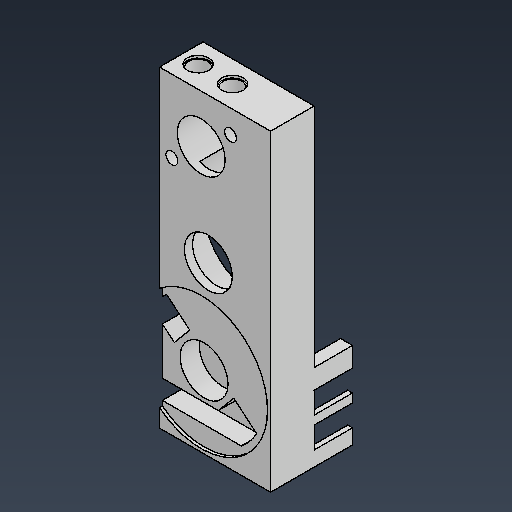
# Autodesk Inventor part: Left_gearbox
Saved by Autodesk Inventor 2026.2 (Build 302298010, 298A)
## iProperties
Created: 2026-04-03
Part Number: Left_gearbox
Material: Generic
Document SubType Name: Modeling
Designer: szymo
Density: 1 g/cm^3
Appearance: Default
Author: szymo
Autodesk Inventor part; units mm, degrees
(part 1 of 2)
ref_plane "YZ Plane" through (0, 0, 0) normal (1, 0, 0) x (0, 1, 0)
ref_plane "XZ Plane" through (0, 0, 0) normal (0, 1, 0) x (-1, 0, 0)
ref_plane "XY Plane" through (0, 0, 0) normal (0, 0, 1) x (1, 0, 0)
ref_plane "Work Plane3" through (-33.4195, -4.4195, -0.6) normal (0, 0, -1) x (-0.5, 0.8660254, 0)
ref_plane "Work Plane4" through (-33.7893, 35.5042, 0.6) normal (0, 0, -1) x (-0.5735764, 0.819152, 0)
sketch "Sketch2" plane through (0, 0, 0) normal (0, 0, 1) x (1, 0, 0)
  circle A0 centre (-8.3716, 60.4381) radius 1.0564 construction
  circle A1 centre (-20.6284, 50.1535) radius 1.0564 construction
  circle A2 centre (-14.5, 55.2958) radius 5
  circle A3 centre (-14.5, 55.2958) radius 13.85 construction
  circle A4 centre (-8.9947, 46.9477) radius 1.25 construction
  arc A5 (-11.5285, 53.3387) -> (-12.3283, 54.22) centre (-15.6066, 50.4414) ccw construction
  arc A6 (-11.1905, 53.4626) -> (-11.5285, 53.3387) centre (-8.9947, 46.9477) ccw construction
  arc A7 (-11.1496, 54.652) -> (-11.1905, 53.4626) centre (-6.206, 53.8864) ccw construction
  arc A8 (-10.7434, 54.7542) -> (-11.1496, 54.652) centre (-8.9947, 46.9477) ccw construction
  arc A9 (-10.1443, 53.7259) -> (-10.7434, 54.7542) centre (-14.7357, 51.7398) ccw construction
  arc A10 (-9.788, 53.7767) -> (-10.1443, 53.7259) centre (-8.9947, 46.9477) ccw construction
  arc A11 (-9.5007, 54.9316) -> (-9.788, 53.7767) centre (-4.8243, 53.1549) ccw construction
  arc A12 (-9.0821, 54.9472) -> (-9.5007, 54.9316) centre (-8.9947, 46.9477) ccw construction
  arc A13 (-8.7099, 53.8168) -> (-9.0821, 54.9472) centre (-13.6139, 52.8287) ccw construction
  arc A14 (-8.3508, 53.7924) -> (-8.7099, 53.8168) centre (-8.9947, 46.9477) ccw construction
  arc A15 (-7.8296, 54.8624) -> (-8.3508, 53.7924) centre (-3.6248, 52.1522) ccw construction
  arc A16 (-7.417, 54.7905) -> (-7.8296, 54.8624) centre (-8.9947, 46.9477) ccw construction
  arc A17 (-7.288, 53.6074) -> (-7.417, 54.7905) centre (-12.2903, 53.6605) ccw construction
  arc A18 (-6.9418, 53.509) -> (-7.288, 53.6074) centre (-8.9947, 46.9477) ccw construction
  arc A19 (-6.2095, 54.4472) -> (-6.9418, 53.509) centre (-2.6601, 50.922) ccw construction
  arc A20 (-5.8209, 54.2911) -> (-6.2095, 54.4472) centre (-8.9947, 46.9477) ccw construction
  arc A21 (-5.9406, 53.1071) -> (-5.8209, 54.2911) centre (-10.8226, 54.199) ccw construction
  arc A22 (-5.6225, 52.9388) -> (-5.9406, 53.1071) centre (-8.9947, 46.9477) ccw construction
  arc A23 (-4.7112, 53.7042) -> (-5.6225, 52.9388) centre (-1.9722, 49.5181) ccw construction
  arc A24 (-4.3634, 53.4708) -> (-4.7112, 53.7042) centre (-8.9947, 46.9477) ccw construction
  arc A25 (-4.7268, 52.3375) -> (-4.3634, 53.4708) centre (-9.275, 54.4206) ccw construction
  arc A26 (-4.4505, 52.1067) -> (-4.7268, 52.3375) centre (-8.9947, 46.9477) ccw construction
  arc A27 (-3.4, 52.666) -> (-4.4505, 52.1067) centre (-1.5913, 48.0019) ccw construction
  arc A28 (-3.1084, 52.3653) -> (-3.4, 52.666) centre (-8.9947, 46.9477) ccw construction
  arc A29 (-3.6994, 51.3323) -> (-3.1084, 52.3653) centre (-7.7151, 54.3155) ccw construction
  arc A30 (-3.4772, 51.0492) -> (-3.6994, 51.3323) centre (-8.9947, 46.9477) ccw construction
  arc A31 (-2.3334, 51.3778) -> (-3.4772, 51.0492) centre (-1.5339, 46.4396) ccw construction
  arc A32 (-2.1106, 51.0231) -> (-2.3334, 51.3778) centre (-8.9947, 46.9477) ccw construction
  arc A33 (-2.9035, 50.1356) -> (-2.1106, 51.0231) centre (-6.2112, 53.8885) ccw construction
  arc A34 (-2.745, 49.8124) -> (-2.9035, 50.1356) centre (-8.9947, 46.9477) ccw construction
  arc A35 (-1.5579, 49.896) -> (-2.745, 49.8124) centre (-1.8025, 44.8995) ccw construction
  arc A36 (-1.4137, 49.5027) -> (-1.5579, 49.896) centre (-8.9947, 46.9477) ccw construction
  arc A37 (-2.3738, 48.7995) -> (-1.4137, 49.5027) centre (-4.829, 53.1581) ccw construction
  arc A38 (-2.286, 48.4504) -> (-2.3738, 48.7995) centre (-8.9947, 46.9477) ccw construction
  arc A39 (-1.1074, 48.2854) -> (-2.286, 48.4504) centre (-2.3855, 43.4489) ccw construction
  arc A40 (-1.0482, 47.8707) -> (-1.1074, 48.2854) centre (-8.9947, 46.9477) ccw construction
  arc A41 (-2.1335, 47.3824) -> (-1.0482, 47.8707) centre (-3.6288, 52.1563) ccw construction
  arc A42 (-2.1202, 47.0227) -> (-2.1335, 47.3824) centre (-8.9947, 46.9477) ccw construction
  arc A43 (-1.0016, 46.6163) -> (-2.1202, 47.0227) centre (-3.2574, 42.1512) ccw construction
  arc A44 (-1.0299, 46.1984) -> (-1.0016, 46.6163) centre (-8.9947, 46.9477) ccw construction
  arc A45 (-2.193, 45.9464) -> (-1.0299, 46.1984) centre (-2.6631, 50.9268) ccw construction
  arc A46 (-2.2548, 45.5918) -> (-2.193, 45.9464) centre (-8.9947, 46.9477) ccw construction
  arc A47 (-1.2452, 44.9616) -> (-2.2548, 45.5918) centre (-4.38, 41.0632) ccw construction
  arc A48 (-1.3597, 44.5588) -> (-1.2452, 44.9616) centre (-8.9947, 46.9477) ccw construction
  arc A49 (-2.5499, 44.5541) -> (-1.3597, 44.5588) centre (-1.9742, 49.5234) ccw construction
  arc A50 (-2.684, 44.2201) -> (-2.5499, 44.5541) centre (-8.9947, 46.9477) ccw construction
  arc A51 (-1.8274, 43.3938) -> (-2.684, 44.2201) centre (-5.7043, 40.2323) ccw construction
  arc A52 (-2.0233, 43.0236) -> (-1.8274, 43.3938) centre (-8.9947, 46.9477) ccw construction
  arc A53 (-3.1883, 43.2665) -> (-2.0233, 43.0236) centre (-1.5921, 48.0075) ccw construction
  arc A54 (-3.3889, 42.9676) -> (-3.1883, 43.2665) centre (-8.9947, 46.9477) ccw construction
  arc A55 (-2.723, 41.9813) -> (-3.3889, 42.9676) centre (-7.1724, 39.6949) ccw construction
  arc A56 (-2.9915, 41.6599) -> (-2.723, 41.9813) centre (-8.9947, 46.9477) ccw construction
  arc A57 (-4.0806, 42.1397) -> (-2.9915, 41.6599) centre (-1.5335, 46.4452) ccw construction
  arc A58 (-4.3389, 41.8891) -> (-4.0806, 42.1397) centre (-8.9947, 46.9477) ccw construction
  arc A59 (-3.8926, 40.7858) -> (-4.3389, 41.8891) centre (-8.7202, 39.4745) ccw construction
  arc A60 (-4.2221, 40.5273) -> (-3.8926, 40.7858) centre (-8.9947, 46.9477) ccw construction
  arc A61 (-5.1876, 41.223) -> (-4.2221, 40.5273) centre (-1.801, 44.9049) ccw construction
  arc A62 (-5.4924, 41.0316) -> (-5.1876, 41.223) centre (-8.9947, 46.9477) ccw construction
  arc A63 (-5.2852, 39.8597) -> (-5.4924, 41.0316) centre (-10.2799, 39.5808) ccw construction
  arc A64 (-5.6612, 39.6753) -> (-5.2852, 39.8597) centre (-8.9947, 46.9477) ccw construction
  arc A65 (-6.461, 40.5566) -> (-5.6612, 39.6753) centre (-2.3829, 43.4539) ccw construction
  arc A66 (-6.799, 40.4327) -> (-6.461, 40.5566) centre (-8.9947, 46.9477) ccw construction
  arc A67 (-6.8399, 39.2433) -> (-6.799, 40.4327) centre (-11.7835, 40.0089) ccw construction
  arc A68 (-7.2461, 39.1411) -> (-6.8399, 39.2433) centre (-8.9947, 46.9477) ccw construction
  arc A69 (-7.8452, 40.1695) -> (-7.2461, 39.1411) centre (-3.2538, 42.1556) ccw construction
  arc A70 (-8.2015, 40.1186) -> (-7.8452, 40.1695) centre (-8.9947, 46.9477) ccw construction
  arc A71 (-8.4888, 38.9637) -> (-8.2015, 40.1186) centre (-13.1652, 40.7404) ccw construction
  arc A72 (-8.9074, 38.9481) -> (-8.4888, 38.9637) centre (-8.9947, 46.9477) ccw construction
  arc A73 (-9.2795, 40.0786) -> (-8.9074, 38.9481) centre (-4.3756, 41.0667) ccw construction
  arc A74 (-9.6387, 40.1029) -> (-9.2795, 40.0786) centre (-8.9947, 46.9477) ccw construction
  arc A75 (-10.1598, 39.033) -> (-9.6387, 40.1029) centre (-14.3646, 41.7431) ccw construction
  arc A76 (-10.5725, 39.1048) -> (-10.1598, 39.033) centre (-8.9947, 46.9477) ccw construction
  arc A77 (-10.7015, 40.2879) -> (-10.5725, 39.1048) centre (-5.6992, 40.2348) ccw construction
  arc A78 (-11.0477, 40.3863) -> (-10.7015, 40.2879) centre (-8.9947, 46.9477) ccw construction
  arc A79 (-11.7799, 39.4481) -> (-11.0477, 40.3863) centre (-15.3294, 42.9733) ccw construction
  arc A80 (-12.1686, 39.6042) -> (-11.7799, 39.4481) centre (-8.9947, 46.9477) ccw construction
  arc A81 (-12.0488, 40.7883) -> (-12.1686, 39.6042) centre (-7.1669, 39.6963) ccw construction
  arc A82 (-12.367, 40.9565) -> (-12.0488, 40.7883) centre (-8.9947, 46.9477) ccw construction
  arc A83 (-13.2783, 40.1911) -> (-12.367, 40.9565) centre (-16.0173, 44.3772) ccw construction
  arc A84 (-13.6261, 40.4246) -> (-13.2783, 40.1911) centre (-8.9947, 46.9477) ccw construction
  arc A85 (-13.2627, 41.5578) -> (-13.6261, 40.4246) centre (-8.7145, 39.4747) ccw construction
  arc A86 (-13.5389, 41.7886) -> (-13.2627, 41.5578) centre (-8.9947, 46.9477) ccw construction
  arc A87 (-14.5895, 41.2294) -> (-13.5389, 41.7886) centre (-16.3982, 45.8935) ccw construction
  arc A88 (-14.8811, 41.53) -> (-14.5895, 41.2294) centre (-8.9947, 46.9477) ccw construction
  arc A89 (-14.29, 42.563) -> (-14.8811, 41.53) centre (-10.2743, 39.5798) ccw construction
  arc A90 (-14.5123, 42.8461) -> (-14.29, 42.563) centre (-8.9947, 46.9477) ccw construction
  arc A91 (-15.6561, 42.5175) -> (-14.5123, 42.8461) centre (-16.4556, 47.4558) ccw construction
  arc A92 (-15.8788, 42.8722) -> (-15.6561, 42.5175) centre (-8.9947, 46.9477) ccw construction
  arc A93 (-15.086, 43.7598) -> (-15.8788, 42.8722) centre (-11.7782, 40.0068) ccw construction
  arc A94 (-15.2445, 44.0829) -> (-15.086, 43.7598) centre (-8.9947, 46.9477) ccw construction
  arc A95 (-16.4316, 43.9993) -> (-15.2445, 44.0829) centre (-16.187, 48.9959) ccw construction
  arc A96 (-16.5757, 44.3926) -> (-16.4316, 43.9993) centre (-8.9947, 46.9477) ccw construction
  arc A97 (-15.6157, 45.0959) -> (-16.5757, 44.3926) centre (-13.1605, 40.7372) ccw construction
  arc A98 (-15.7035, 45.4449) -> (-15.6157, 45.0959) centre (-8.9947, 46.9477) ccw construction
  arc A99 (-16.8821, 45.61) -> (-15.7035, 45.4449) centre (-15.6039, 50.4465) ccw construction
  arc A100 (-16.9413, 46.0246) -> (-16.8821, 45.61) centre (-8.9947, 46.9477) ccw construction
  arc A101 (-15.856, 46.5129) -> (-16.9413, 46.0246) centre (-14.3607, 41.739) ccw construction
  arc A102 (-15.8693, 46.8726) -> (-15.856, 46.5129) centre (-8.9947, 46.9477) ccw construction
  arc A103 (-16.9879, 47.2791) -> (-15.8693, 46.8726) centre (-14.7321, 51.7441) ccw construction
  arc A104 (-16.9596, 47.6969) -> (-16.9879, 47.2791) centre (-8.9947, 46.9477) ccw construction
  arc A105 (-15.7964, 47.9489) -> (-16.9596, 47.6969) centre (-15.3264, 42.9685) ccw construction
  arc A106 (-15.7347, 48.3035) -> (-15.7964, 47.9489) centre (-8.9947, 46.9477) ccw construction
  arc A107 (-16.7443, 48.9337) -> (-15.7347, 48.3035) centre (-13.6095, 52.8322) ccw construction
  arc A108 (-16.6297, 49.3365) -> (-16.7443, 48.9337) centre (-8.9947, 46.9477) ccw construction
  arc A109 (-15.4396, 49.3412) -> (-16.6297, 49.3365) centre (-16.0153, 44.3719) ccw construction
  arc A110 (-15.3055, 49.6752) -> (-15.4396, 49.3412) centre (-8.9947, 46.9477) ccw construction
  arc A111 (-16.162, 50.5015) -> (-15.3055, 49.6752) centre (-12.2852, 53.663) ccw construction
  arc A112 (-15.9662, 50.8717) -> (-16.162, 50.5015) centre (-8.9947, 46.9477) ccw construction
  arc A113 (-14.8012, 50.6289) -> (-15.9662, 50.8717) centre (-16.3974, 45.8878) ccw construction
  arc A114 (-14.6005, 50.9277) -> (-14.8012, 50.6289) centre (-8.9947, 46.9477) ccw construction
  arc A115 (-15.2665, 51.914) -> (-14.6005, 50.9277) centre (-10.817, 54.2004) ccw construction
  arc A116 (-14.998, 52.2355) -> (-15.2665, 51.914) centre (-8.9947, 46.9477) ccw construction
  arc A117 (-13.9089, 51.7556) -> (-14.998, 52.2355) centre (-16.456, 47.4501) ccw construction
  arc A118 (-13.6505, 52.0062) -> (-13.9089, 51.7556) centre (-8.9947, 46.9477) ccw construction
  arc A119 (-14.0969, 53.1095) -> (-13.6505, 52.0062) centre (-9.2693, 54.4208) ccw construction
  arc A120 (-13.7674, 53.368) -> (-14.0969, 53.1095) centre (-8.9947, 46.9477) ccw construction
  arc A121 (-12.8019, 52.6723) -> (-13.7674, 53.368) centre (-16.1885, 48.9904) ccw construction
  arc A122 (-12.4971, 52.8637) -> (-12.8019, 52.6723) centre (-8.9947, 46.9477) ccw construction
  arc A123 (-12.7043, 54.0356) -> (-12.4971, 52.8637) centre (-7.7095, 54.3146) ccw construction
  arc A124 (-12.3283, 54.22) -> (-12.7043, 54.0356) centre (-8.9947, 46.9477) ccw construction
  circle A125 centre (-13, 35.0012) radius 5
  arc A126 (-19.3741, 42.1797) -> (-18.7931, 40.8751) centre (-13.6387, 43.9522) ccw construction
  arc A127 (-18.7931, 40.8751) -> (-19.0926, 40.5639) centre (-13, 35.0012) ccw construction
  arc A128 (-19.0926, 40.5639) -> (-20.4186, 41.0942) centre (-21.969, 35.2948) ccw construction
  arc A129 (-20.4186, 41.0942) -> (-20.7273, 40.6976) centre (-13, 35.0012) ccw construction
  arc A130 (-20.7273, 40.6976) -> (-19.8878, 39.5423) centre (-15.4858, 43.6238) ccw construction
  arc A131 (-19.8878, 39.5423) -> (-20.116, 39.1756) centre (-13, 35.0012) ccw construction
  arc A132 (-20.116, 39.1756) -> (-21.5233, 39.4186) centre (-21.8341, 33.4236) ccw construction
  arc A133 (-21.5233, 39.4186) -> (-21.7428, 38.9665) centre (-13, 35.0012) ccw construction
  arc A134 (-21.7428, 38.9665) -> (-20.6814, 38.011) centre (-17.2242, 42.9186) ccw construction
  arc A135 (-20.6814, 38.011) -> (-20.8284, 37.6049) centre (-13, 35.0012) ccw construction
  arc A136 (-20.8284, 37.6049) -> (-22.2555, 37.55) centre (-21.313, 31.6214) ccw construction
  arc A137 (-22.2555, 37.55) -> (-22.3762, 37.0621) centre (-13, 35.0012) ccw construction
  arc A138 (-22.3762, 37.0621) -> (-21.1393, 36.3482) centre (-18.778, 41.8673) ccw construction
  arc A139 (-21.1393, 36.3482) -> (-21.1986, 35.9204) centre (-13, 35.0012) ccw construction
  arc A140 (-21.1986, 35.9204) -> (-22.5831, 35.57) centre (-20.4287, 29.9669) ccw construction
  arc A141 (-22.5831, 35.57) -> (-22.5998, 35.0677) centre (-13, 35.0012) ccw construction
  arc A142 (-22.5998, 35.0677) -> (-21.2415, 34.6265) centre (-20.0793, 40.516) ccw construction
  arc A143 (-21.2415, 34.6265) -> (-21.2106, 34.1957) centre (-13, 35.0012) ccw construction
  arc A144 (-21.2106, 34.1957) -> (-22.492, 33.5651) centre (-19.2196, 28.5324) ccw construction
  arc A145 (-22.492, 33.5651) -> (-22.4038, 33.0703) centre (-13, 35.0012) ccw construction
  arc A146 (-22.4038, 33.0703) -> (-20.9835, 32.9212) centre (-21.0712, 38.9236) ccw construction
  arc A147 (-20.9835, 32.9212) -> (-20.8637, 32.5062) centre (-13, 35.0012) ccw construction
  arc A148 (-20.8637, 32.5062) -> (-21.986, 31.623) centre (-17.7388, 27.3806) ccw construction
  arc A149 (-21.986, 31.623) -> (-21.7969, 31.1574) centre (-13, 35.0012) ccw construction
  arc A150 (-21.7969, 31.1574) -> (-20.3766, 31.3068) centre (-21.7103, 37.1598) ccw construction
  arc A151 (-20.3766, 31.3068) -> (-20.1731, 30.9258) centre (-13, 35.0012) ccw construction
  arc A152 (-20.1731, 30.9258) -> (-21.0873, 29.8285) centre (-16.0508, 26.5619) ccw construction
  arc A153 (-21.0873, 29.8285) -> (-20.8055, 29.4124) centre (-13, 35.0012) ccw construction
  arc A154 (-20.8055, 29.4124) -> (-19.4473, 29.8538) centre (-21.9688, 35.3016) ccw construction
  arc A155 (-19.4473, 29.8538) -> (-19.169, 29.5235) centre (-13, 35.0012) ccw construction
  arc A156 (-19.169, 29.5235) -> (-19.8351, 28.2601) centre (-14.2295, 26.112) ccw construction
  arc A157 (-19.8351, 28.2601) -> (-19.4729, 27.9117) centre (-13, 35.0012) ccw construction
  arc A158 (-19.4729, 27.9117) -> (-18.2362, 28.6259) centre (-21.8352, 33.4304) ccw construction
  arc A159 (-18.2362, 28.6259) -> (-17.8953, 28.3605) centre (-13, 35.0012) ccw construction
  arc A160 (-17.8953, 28.3605) -> (-18.2842, 26.9864) centre (-12.3545, 26.0506) ccw construction
  arc A161 (-18.2842, 26.9864) -> (-17.8575, 26.7208) centre (-13, 35.0012) ccw construction
  arc A162 (-17.8575, 26.7208) -> (-16.7962, 27.6765) centre (-21.3156, 31.6277) ccw construction
  arc A163 (-16.7962, 27.6765) -> (-16.4077, 27.4879) centre (-13, 35.0012) ccw construction
  arc A164 (-16.4077, 27.4879) -> (-16.5023, 26.0629) centre (-10.5077, 26.3804) ccw construction
  arc A165 (-16.5023, 26.0629) -> (-16.0297, 25.8918) centre (-13, 35.0012) ccw construction
  arc A166 (-16.0297, 25.8918) -> (-15.1904, 27.0473) centre (-20.4325, 29.9725) ccw construction
  arc A167 (-15.1904, 27.0473) -> (-14.7711, 26.9436) centre (-13, 35.0012) ccw construction
  arc A168 (-14.7711, 26.9436) -> (-14.5674, 25.53) centre (-8.7698, 27.087) ccw construction
  arc A169 (-14.5674, 25.53) -> (-14.0696, 25.461) centre (-13, 35.0012) ccw construction
  arc A170 (-14.0696, 25.461) -> (-13.4888, 26.7657) centre (-19.2245, 28.5371) ccw construction
  arc A171 (-13.4888, 26.7657) -> (-13.0571, 26.7514) centre (-13, 35.0012) ccw construction
  arc A172 (-13.0571, 26.7514) -> (-12.564, 25.4111) centre (-7.2168, 28.1395) ccw construction
  arc A173 (-12.564, 25.4111) -> (-12.0627, 25.4471) centre (-13, 35.0012) ccw construction
  arc A174 (-12.0627, 25.4471) -> (-11.7659, 26.844) centre (-17.7446, 27.3842) ccw construction
  arc A175 (-11.7659, 26.844) -> (-11.3407, 26.9198) centre (-13, 35.0012) ccw construction
  arc A176 (-11.3407, 26.9198) -> (-10.5796, 25.7113) centre (-5.9165, 29.4918) ccw construction
  arc A177 (-10.5796, 25.7113) -> (-10.0967, 25.8507) centre (-13, 35.0012) ccw construction
  arc A178 (-10.0967, 25.8507) -> (-10.0969, 27.2789) centre (-16.0572, 26.5642) ccw construction
  arc A179 (-10.0969, 27.2789) -> (-9.6967, 27.4414) centre (-13, 35.0012) ccw construction
  arc A180 (-9.6967, 27.4414) -> (-8.701, 26.4176) centre (-4.9258, 31.0849) ccw construction
  arc A181 (-8.701, 26.4176) -> (-8.2577, 26.6543) centre (-13, 35.0012) ccw construction
  arc A182 (-8.2577, 26.6543) -> (-8.5548, 28.0512) centre (-14.2363, 26.113) ccw construction
  arc A183 (-8.5548, 28.0512) -> (-8.1971, 28.2934) centre (-13, 35.0012) ccw construction
  arc A184 (-8.1971, 28.2934) -> (-7.0103, 27.4989) centre (-4.288, 32.8492) ccw construction
  arc A185 (-7.0103, 27.4989) -> (-6.6259, 27.8227) centre (-13, 35.0012) ccw construction
  arc A186 (-6.6259, 27.8227) -> (-7.2069, 29.1273) centre (-12.3613, 26.0502) ccw construction
  arc A187 (-7.2069, 29.1273) -> (-6.9074, 29.4385) centre (-13, 35.0012) ccw construction
  arc A188 (-6.9074, 29.4385) -> (-5.5814, 28.9082) centre (-4.031, 34.7076) ccw construction
  arc A189 (-5.5814, 28.9082) -> (-5.2727, 29.3048) centre (-13, 35.0012) ccw construction
  arc A190 (-5.2727, 29.3048) -> (-6.1122, 30.4601) centre (-10.5142, 26.3786) ccw construction
  arc A191 (-6.1122, 30.4601) -> (-5.884, 30.8268) centre (-13, 35.0012) ccw construction
  arc A192 (-5.884, 30.8268) -> (-4.4767, 30.5838) centre (-4.1659, 36.5788) ccw construction
  arc A193 (-4.4767, 30.5838) -> (-4.2572, 31.0359) centre (-13, 35.0012) ccw construction
  arc A194 (-4.2572, 31.0359) -> (-5.3186, 31.9914) centre (-8.7758, 27.0838) ccw construction
  arc A195 (-5.3186, 31.9914) -> (-5.1716, 32.3975) centre (-13, 35.0012) ccw construction
  arc A196 (-5.1716, 32.3975) -> (-3.7445, 32.4524) centre (-4.687, 38.381) ccw construction
  arc A197 (-3.7445, 32.4524) -> (-3.6238, 32.9403) centre (-13, 35.0012) ccw construction
  arc A198 (-3.6238, 32.9403) -> (-4.8607, 33.6542) centre (-7.222, 28.1351) ccw construction
  arc A199 (-4.8607, 33.6542) -> (-4.8014, 34.082) centre (-13, 35.0012) ccw construction
  arc A200 (-4.8014, 34.082) -> (-3.4169, 34.4324) centre (-5.5713, 40.0355) ccw construction
  arc A201 (-3.4169, 34.4324) -> (-3.4002, 34.9347) centre (-13, 35.0012) ccw construction
  arc A202 (-3.4002, 34.9347) -> (-4.7585, 35.3759) centre (-5.9207, 29.4864) ccw construction
  arc A203 (-4.7585, 35.3759) -> (-4.7894, 35.8067) centre (-13, 35.0012) ccw construction
  arc A204 (-4.7894, 35.8067) -> (-3.508, 36.4373) centre (-6.7804, 41.47) ccw construction
  arc A205 (-3.508, 36.4373) -> (-3.5962, 36.9321) centre (-13, 35.0012) ccw construction
  arc A206 (-3.5962, 36.9321) -> (-5.0165, 37.0812) centre (-4.9288, 31.0788) ccw construction
  arc A207 (-5.0165, 37.0812) -> (-5.1363, 37.4962) centre (-13, 35.0012) ccw construction
  arc A208 (-5.1363, 37.4962) -> (-4.014, 38.3794) centre (-8.2612, 42.6218) ccw construction
  arc A209 (-4.014, 38.3794) -> (-4.2031, 38.845) centre (-13, 35.0012) ccw construction
  arc A210 (-4.2031, 38.845) -> (-5.6234, 38.6956) centre (-4.2897, 32.8426) ccw construction
  arc A211 (-5.6234, 38.6956) -> (-5.8269, 39.0766) centre (-13, 35.0012) ccw construction
  arc A212 (-5.8269, 39.0766) -> (-4.9127, 40.1739) centre (-9.9492, 43.4405) ccw construction
  arc A213 (-4.9127, 40.1739) -> (-5.1945, 40.59) centre (-13, 35.0012) ccw construction
  arc A214 (-5.1945, 40.59) -> (-6.5527, 40.1486) centre (-4.0312, 34.7008) ccw construction
  arc A215 (-6.5527, 40.1486) -> (-6.831, 40.4789) centre (-13, 35.0012) ccw construction
  arc A216 (-6.831, 40.4789) -> (-6.1649, 41.7423) centre (-11.7705, 43.8904) ccw construction
  arc A217 (-6.1649, 41.7423) -> (-6.5271, 42.0907) centre (-13, 35.0012) ccw construction
  arc A218 (-6.5271, 42.0907) -> (-7.7638, 41.3765) centre (-4.1648, 36.572) ccw construction
  arc A219 (-7.7638, 41.3765) -> (-8.1047, 41.6418) centre (-13, 35.0012) ccw construction
  arc A220 (-8.1047, 41.6418) -> (-7.7158, 43.016) centre (-13.6455, 43.9518) ccw construction
  arc A221 (-7.7158, 43.016) -> (-8.1425, 43.2816) centre (-13, 35.0012) ccw construction
  arc A222 (-8.1425, 43.2816) -> (-9.2038, 42.3259) centre (-4.6844, 38.3747) ccw construction
  arc A223 (-9.2038, 42.3259) -> (-9.5923, 42.5145) centre (-13, 35.0012) ccw construction
  arc A224 (-9.5923, 42.5145) -> (-9.4977, 43.9395) centre (-15.4923, 43.622) ccw construction
  arc A225 (-9.4977, 43.9395) -> (-9.9703, 44.1106) centre (-13, 35.0012) ccw construction
  arc A226 (-9.9703, 44.1106) -> (-10.8096, 42.9551) centre (-5.5675, 40.0299) ccw construction
  arc A227 (-10.8096, 42.9551) -> (-11.2289, 43.0588) centre (-13, 35.0012) ccw construction
  arc A228 (-11.2289, 43.0588) -> (-11.4326, 44.4724) centre (-17.2302, 42.9154) ccw construction
  arc A229 (-11.4326, 44.4724) -> (-11.9304, 44.5414) centre (-13, 35.0012) ccw construction
  arc A230 (-11.9304, 44.5414) -> (-12.5112, 43.2367) centre (-6.7755, 41.4653) ccw construction
  arc A231 (-12.5112, 43.2367) -> (-12.9429, 43.251) centre (-13, 35.0012) ccw construction
  arc A232 (-12.9429, 43.251) -> (-13.436, 44.5913) centre (-18.7832, 41.8629) ccw construction
  arc A233 (-13.436, 44.5913) -> (-13.9373, 44.5553) centre (-13, 35.0012) ccw construction
  arc A234 (-13.9373, 44.5553) -> (-14.2341, 43.1584) centre (-8.2554, 42.6182) ccw construction
  arc A235 (-14.2341, 43.1584) -> (-14.6593, 43.0826) centre (-13, 35.0012) ccw construction
  arc A236 (-14.6593, 43.0826) -> (-15.4204, 44.2911) centre (-20.0835, 40.5106) ccw construction
  arc A237 (-15.4204, 44.2911) -> (-15.9033, 44.1517) centre (-13, 35.0012) ccw construction
  arc A238 (-15.9033, 44.1517) -> (-15.9031, 42.7235) centre (-9.9428, 43.4382) ccw construction
  arc A239 (-15.9031, 42.7235) -> (-16.3033, 42.561) centre (-13, 35.0012) ccw construction
  arc A240 (-16.3033, 42.561) -> (-17.299, 43.5848) centre (-21.0742, 38.9175) ccw construction
  arc A241 (-17.299, 43.5848) -> (-17.7423, 43.3481) centre (-13, 35.0012) ccw construction
  arc A242 (-17.7423, 43.3481) -> (-17.4452, 41.9512) centre (-11.7637, 43.8894) ccw construction
  arc A243 (-17.4452, 41.9512) -> (-17.8029, 41.709) centre (-13, 35.0012) ccw construction
  arc A244 (-17.8029, 41.709) -> (-18.9897, 42.5035) centre (-21.712, 37.1532) ccw construction
  arc A245 (-18.9897, 42.5035) -> (-19.3741, 42.1797) centre (-13, 35.0012) ccw construction
  line L0 (0, 0) -> (-23.2, 0)
  line L1 (-23.2, 0) -> (-23.2, 65.2958)
  line L2 (-23.2, 65.2958) -> (0, 65.2958)
  line L3 (0, 65.2958) -> (0, 0)
  circle A246 centre (-13, 35.0012) radius 9.6
  circle A247 centre (-8.9947, 46.9477) radius 8
  line L4 (-14.5, 65.2958) -> (-14.5, 55.2958) construction
  circle A248 centre (-14.5, 55.2958) radius 14.5 construction
  circle A249 centre (-14.5, 14.5) radius 14.5 construction
  line L5 (-14.5, 65.2958) -> (-14.5, 69.7958) construction
  circle A250 centre (-8.9947, 46.9477) radius 8.4
  circle A251 centre (-13, 35.0012) radius 10
  line L6 (-20.7032, 16.4416) -> (-25.4891, 20.4574)
  arc A252 (-22.2751, 24.2876) -> (-25.4891, 20.4574) centre (-14.5, 14.5) ccw
  line L7 (-22.2751, 24.2876) -> (-17.4893, 20.2718)
  arc A253 (-17.4893, 20.2718) -> (-20.7032, 16.4416) centre (-14.5, 14.5) ccw construction
  line L8 (-8.2968, 12.5584) -> (-3.5109, 8.5426)
  arc A254 (-6.7249, 4.7124) -> (-3.5109, 8.5426) centre (-14.5, 14.5) ccw
  line L9 (-6.7249, 4.7124) -> (-11.5107, 8.7282)
  arc A255 (-11.5107, 8.7282) -> (-8.2968, 12.5584) centre (-14.5, 14.5) ccw construction
  line L10 (-17.4893, 20.2718) -> (-20.7032, 16.4416)
  line L11 (-8.2968, 12.5584) -> (-11.5107, 8.7282)
  line L12 (-11.5107, 8.7282) -> (-23.2, 8.7282)
  line L13 (-6.7249, 4.7124) -> (-23.2, 4.7124)
  line L14 (-20.7032, 16.4416) -> (-25.4891, 20.4574)
  arc A256 (-22.2751, 24.2876) -> (-25.4891, 20.4574) centre (-14.5, 14.5) ccw
  line L15 (-22.2751, 24.2876) -> (-17.4893, 20.2718)
  arc A257 (-17.4893, 20.2718) -> (-20.7032, 16.4416) centre (-14.5, 14.5) ccw
  arc A258 (-6.7249, 4.7124) -> (-3.5109, 8.5426) centre (-14.5, 14.5) ccw
  line L16 (-3.5109, 8.5426) -> (-8.2968, 12.5584)
  arc A259 (-11.5107, 8.7282) -> (-8.2968, 12.5584) centre (-14.5, 14.5) ccw
  line L17 (-11.5107, 8.7282) -> (-6.7249, 4.7124)
  line L18 (-19.1651, 20.3726) -> (-22.2701, 22.978)
  arc A260 (-22.2701, 22.978) -> (-24.1984, 20.6798) centre (-14.5, 14.5) ccw
  line L19 (-24.1984, 20.6798) -> (-21.0934, 18.0744)
  arc A261 (-19.1651, 20.3726) -> (-21.0934, 18.0744) centre (-14.5, 14.5) ccw
  arc A262 (-6.7299, 6.022) -> (-4.8016, 8.3202) centre (-14.5, 14.5) ccw
  line L20 (-4.8016, 8.3202) -> (-7.9066, 10.9256)
  arc A263 (-9.8349, 8.6274) -> (-7.9066, 10.9256) centre (-14.5, 14.5) ccw
  line L21 (-9.8349, 8.6274) -> (-6.7299, 6.022)
  circle A264 centre (-14.5, 14.5) radius 5
  circle A265 centre (-14.5, 14.5) radius 13.85
  point P0 (-23.2, 5.021)
  point P1 (-23.2, 20.1674)
  point P2 (-16.4204, 43.9712)
  point P3 (-16.1285, 50.5685)
  point P4 (-9.5133, 54.9308)
  point P5 (-4.8639, 40.0967)
  point P6 (-16.9313, 44.196)
  point P7 (-16.5028, 50.7145)
  point P8 (-9.5001, 55.3324)
  point P9 (-4.3207, 39.9681)
  point P10 (-23.2, 23.7912)
  point P11 (-3.7958, 23.2888)
  point P12 (-4.6587, 39.7533)
  point P13 (-9.4902, 38.5623)
  point P14 (-13.6539, 39.9582)
  point P15 (-16.7911, 43.8209)
  point P16 (-23.2, 23.4755)
  point P17 (-23.2, 18.5366)
  point P18 (-16.5599, 44.3461)
  point P19 (-4.5266, 40.3117)
  point P20 (-23.2, 22.4097)
  point P21 (-23.2, 23.4755)
  point P22 (-23.2, 3.7235)
  point P23 (-23.2, 25.2765)
extrude "Extrusion3" add sketch "Sketch2" along normal up to surface (0.6 mm away) contours A2 A250 A251 A247 | A2 A250 A251 A265 L1 L2 L3 L0 | A247 A251 A2 | A2 A247 A251 A250 | A251 A247 A246 A250 | A250 A246 A265 A251 | A251 A265 A246 A250 | A250 A246 A247 A251 | A251 A247 A246 | A250 A125 A246 A265 | A246 A247 A125 A250 | A250 A125 A247 A246 | A246 A247 A125
extrude "Extrusion4" add sketch "Sketch2" against normal blind 1.1 contours A2 A250 A251 A247 | A2 A250 A251 A265 L1 L2 L3 L0 | A247 A251 A2 | A2 A247 A251 A250 | A251 A247 A246 A250 | A250 A246 A265 A251 | A251 A265 A246 A250 | A250 A246 A247 A251 | A251 A247 A246 | A250 A125 A246 A265 | A246 A247 A125 A250 | A265 A246 A251 | A251 A265 L1 L13 A254 L8 L11 L12 L6 L10 L7 A252 | A250 A125 A247 A246 | A246 A247 A125 | A265 A246
extrude "Extrusion5" add sketch "Sketch2" against normal blind 4 contours A2 A250 A251 A265 L1 L2 L3 L0 | A251 A265 L1 L13 A254 L8 L11 L12 L6 L10 L7 A252
ref_plane "Work Plane5" through (0, -2.774, -4) normal (0, 0, 1) x (-1, 0, 0)
sketch "Sketch3" plane through (0, -2.774, -4) normal (0, 0, 1) x (-1, 0, 0)
  line L0 (0, -2.774) -> (23.2, -2.774)
  line L1 (23.2, -2.774) -> (23.2, -68.0698)
  line L2 (23.2, -68.0698) -> (0, -68.0698)
  line L3 (0, -68.0698) -> (0, -2.774)
  circle A0 centre (8.9947, -49.7216) radius 1.25 construction
  arc A1 (11.5285, -56.1127) -> (12.3283, -56.994) centre (15.6066, -53.2154) ccw construction
  arc A2 (11.1905, -56.2365) -> (11.5285, -56.1127) centre (8.9947, -49.7216) ccw construction
  arc A3 (11.1496, -57.4259) -> (11.1905, -56.2365) centre (6.206, -56.6603) ccw construction
  arc A4 (10.7434, -57.5282) -> (11.1496, -57.4259) centre (8.9947, -49.7216) ccw construction
  arc A5 (10.1443, -56.4998) -> (10.7434, -57.5282) centre (14.7357, -54.5137) ccw construction
  arc A6 (9.788, -56.5507) -> (10.1443, -56.4998) centre (8.9947, -49.7216) ccw construction
  arc A7 (9.5007, -57.7056) -> (9.788, -56.5507) centre (4.8243, -55.9289) ccw construction
  arc A8 (9.0821, -57.7211) -> (9.5007, -57.7056) centre (8.9947, -49.7216) ccw construction
  arc A9 (8.7099, -56.5907) -> (9.0821, -57.7211) centre (13.6139, -55.6026) ccw construction
  arc A10 (8.3508, -56.5664) -> (8.7099, -56.5907) centre (8.9947, -49.7216) ccw construction
  arc A11 (7.8296, -57.6363) -> (8.3508, -56.5664) centre (3.6248, -54.9261) ccw construction
  arc A12 (7.417, -57.5645) -> (7.8296, -57.6363) centre (8.9947, -49.7216) ccw construction
  arc A13 (7.288, -56.3814) -> (7.417, -57.5645) centre (12.2903, -56.4345) ccw construction
  arc A14 (6.9418, -56.2829) -> (7.288, -56.3814) centre (8.9947, -49.7216) ccw construction
  arc A15 (6.2095, -57.2211) -> (6.9418, -56.2829) centre (2.6601, -53.6959) ccw construction
  arc A16 (5.8209, -57.0651) -> (6.2095, -57.2211) centre (8.9947, -49.7216) ccw construction
  arc A17 (5.9406, -55.881) -> (5.8209, -57.0651) centre (10.8226, -56.973) ccw construction
  arc A18 (5.6225, -55.7127) -> (5.9406, -55.881) centre (8.9947, -49.7216) ccw construction
  arc A19 (4.7112, -56.4782) -> (5.6225, -55.7127) centre (1.9722, -52.2921) ccw construction
  arc A20 (4.3634, -56.2447) -> (4.7112, -56.4782) centre (8.9947, -49.7216) ccw construction
  arc A21 (4.7268, -55.1114) -> (4.3634, -56.2447) centre (9.275, -57.1945) ccw construction
  arc A22 (4.4505, -54.8807) -> (4.7268, -55.1114) centre (8.9947, -49.7216) ccw construction
  arc A23 (3.4, -55.4399) -> (4.4505, -54.8807) centre (1.5913, -50.7758) ccw construction
  arc A24 (3.1084, -55.1393) -> (3.4, -55.4399) centre (8.9947, -49.7216) ccw construction
  arc A25 (3.6994, -54.1063) -> (3.1084, -55.1393) centre (7.7151, -57.0895) ccw construction
  arc A26 (3.4772, -53.8231) -> (3.6994, -54.1063) centre (8.9947, -49.7216) ccw construction
  arc A27 (2.3334, -54.1517) -> (3.4772, -53.8231) centre (1.5339, -49.2135) ccw construction
  arc A28 (2.1106, -53.797) -> (2.3334, -54.1517) centre (8.9947, -49.7216) ccw construction
  arc A29 (2.9035, -52.9095) -> (2.1106, -53.797) centre (6.2112, -56.6624) ccw construction
  arc A30 (2.745, -52.5864) -> (2.9035, -52.9095) centre (8.9947, -49.7216) ccw construction
  arc A31 (1.5579, -52.67) -> (2.745, -52.5864) centre (1.8025, -47.6734) ccw construction
  arc A32 (1.4137, -52.2767) -> (1.5579, -52.67) centre (8.9947, -49.7216) ccw construction
  arc A33 (2.3738, -51.5734) -> (1.4137, -52.2767) centre (4.829, -55.932) ccw construction
  arc A34 (2.286, -51.2244) -> (2.3738, -51.5734) centre (8.9947, -49.7216) ccw construction
  arc A35 (1.1074, -51.0593) -> (2.286, -51.2244) centre (2.3855, -46.2228) ccw construction
  arc A36 (1.0482, -50.6447) -> (1.1074, -51.0593) centre (8.9947, -49.7216) ccw construction
  arc A37 (2.1335, -50.1564) -> (1.0482, -50.6447) centre (3.6288, -54.9302) ccw construction
  arc A38 (2.1202, -49.7967) -> (2.1335, -50.1564) centre (8.9947, -49.7216) ccw construction
  arc A39 (1.0016, -49.3902) -> (2.1202, -49.7967) centre (3.2574, -44.9251) ccw construction
  arc A40 (1.0299, -48.9723) -> (1.0016, -49.3902) centre (8.9947, -49.7216) ccw construction
  arc A41 (2.193, -48.7204) -> (1.0299, -48.9723) centre (2.6631, -53.7008) ccw construction
  arc A42 (2.2548, -48.3658) -> (2.193, -48.7204) centre (8.9947, -49.7216) ccw construction
  arc A43 (1.2452, -47.7356) -> (2.2548, -48.3658) centre (4.38, -43.8371) ccw construction
  arc A44 (1.3597, -47.3327) -> (1.2452, -47.7356) centre (8.9947, -49.7216) ccw construction
  arc A45 (2.5499, -47.3281) -> (1.3597, -47.3327) centre (1.9742, -52.2974) ccw construction
  arc A46 (2.684, -46.9941) -> (2.5499, -47.3281) centre (8.9947, -49.7216) ccw construction
  arc A47 (1.8274, -46.1678) -> (2.684, -46.9941) centre (5.7043, -43.0062) ccw construction
  arc A48 (2.0233, -45.7975) -> (1.8274, -46.1678) centre (8.9947, -49.7216) ccw construction
  arc A49 (3.1883, -46.0404) -> (2.0233, -45.7975) centre (1.5921, -50.7814) ccw construction
  arc A50 (3.3889, -45.7416) -> (3.1883, -46.0404) centre (8.9947, -49.7216) ccw construction
  arc A51 (2.723, -44.7553) -> (3.3889, -45.7416) centre (7.1724, -42.4689) ccw construction
  arc A52 (2.9915, -44.4338) -> (2.723, -44.7553) centre (8.9947, -49.7216) ccw construction
  arc A53 (4.0806, -44.9136) -> (2.9915, -44.4338) centre (1.5335, -49.2192) ccw construction
  arc A54 (4.3389, -44.663) -> (4.0806, -44.9136) centre (8.9947, -49.7216) ccw construction
  arc A55 (3.8926, -43.5598) -> (4.3389, -44.663) centre (8.7202, -42.2485) ccw construction
  arc A56 (4.2221, -43.3012) -> (3.8926, -43.5598) centre (8.9947, -49.7216) ccw construction
  arc A57 (5.1876, -43.997) -> (4.2221, -43.3012) centre (1.801, -47.6789) ccw construction
  arc A58 (5.4924, -43.8056) -> (5.1876, -43.997) centre (8.9947, -49.7216) ccw construction
  arc A59 (5.2852, -42.6337) -> (5.4924, -43.8056) centre (10.2799, -42.3547) ccw construction
  arc A60 (5.6612, -42.4492) -> (5.2852, -42.6337) centre (8.9947, -49.7216) ccw construction
  arc A61 (6.461, -43.3305) -> (5.6612, -42.4492) centre (2.3829, -46.2278) ccw construction
  arc A62 (6.799, -43.2067) -> (6.461, -43.3305) centre (8.9947, -49.7216) ccw construction
  arc A63 (6.8399, -42.0173) -> (6.799, -43.2067) centre (11.7835, -42.7829) ccw construction
  arc A64 (7.2461, -41.9151) -> (6.8399, -42.0173) centre (8.9947, -49.7216) ccw construction
  arc A65 (7.8452, -42.9434) -> (7.2461, -41.9151) centre (3.2538, -44.9295) ccw construction
  arc A66 (8.2015, -42.8925) -> (7.8452, -42.9434) centre (8.9947, -49.7216) ccw construction
  arc A67 (8.4888, -41.7376) -> (8.2015, -42.8925) centre (13.1652, -43.5143) ccw construction
  arc A68 (8.9074, -41.7221) -> (8.4888, -41.7376) centre (8.9947, -49.7216) ccw construction
  arc A69 (9.2795, -42.8525) -> (8.9074, -41.7221) centre (4.3756, -43.8406) ccw construction
  arc A70 (9.6387, -42.8768) -> (9.2795, -42.8525) centre (8.9947, -49.7216) ccw construction
  arc A71 (10.1598, -41.8069) -> (9.6387, -42.8768) centre (14.3646, -44.5171) ccw construction
  arc A72 (10.5725, -41.8787) -> (10.1598, -41.8069) centre (8.9947, -49.7216) ccw construction
  arc A73 (10.7015, -43.0618) -> (10.5725, -41.8787) centre (5.6992, -43.0087) ccw construction
  arc A74 (11.0477, -43.1603) -> (10.7015, -43.0618) centre (8.9947, -49.7216) ccw construction
  arc A75 (11.7799, -42.2221) -> (11.0477, -43.1603) centre (15.3294, -45.7473) ccw construction
  arc A76 (12.1686, -42.3781) -> (11.7799, -42.2221) centre (8.9947, -49.7216) ccw construction
  arc A77 (12.0488, -43.5622) -> (12.1686, -42.3781) centre (7.1669, -42.4703) ccw construction
  arc A78 (12.367, -43.7305) -> (12.0488, -43.5622) centre (8.9947, -49.7216) ccw construction
  arc A79 (13.2783, -42.9651) -> (12.367, -43.7305) centre (16.0173, -47.1512) ccw construction
  arc A80 (13.6261, -43.1985) -> (13.2783, -42.9651) centre (8.9947, -49.7216) ccw construction
  arc A81 (13.2627, -44.3318) -> (13.6261, -43.1985) centre (8.7145, -42.2487) ccw construction
  arc A82 (13.5389, -44.5626) -> (13.2627, -44.3318) centre (8.9947, -49.7216) ccw construction
  arc A83 (14.5895, -44.0033) -> (13.5389, -44.5626) centre (16.3982, -48.6674) ccw construction
  arc A84 (14.8811, -44.304) -> (14.5895, -44.0033) centre (8.9947, -49.7216) ccw construction
  arc A85 (14.29, -45.3369) -> (14.8811, -44.304) centre (10.2743, -42.3537) ccw construction
  arc A86 (14.5123, -45.6201) -> (14.29, -45.3369) centre (8.9947, -49.7216) ccw construction
  arc A87 (15.6561, -45.2915) -> (14.5123, -45.6201) centre (16.4556, -50.2297) ccw construction
  arc A88 (15.8788, -45.6462) -> (15.6561, -45.2915) centre (8.9947, -49.7216) ccw construction
  arc A89 (15.086, -46.5337) -> (15.8788, -45.6462) centre (11.7782, -42.7808) ccw construction
  arc A90 (15.2445, -46.8569) -> (15.086, -46.5337) centre (8.9947, -49.7216) ccw construction
  arc A91 (16.4316, -46.7733) -> (15.2445, -46.8569) centre (16.187, -51.7698) ccw construction
  arc A92 (16.5757, -47.1665) -> (16.4316, -46.7733) centre (8.9947, -49.7216) ccw construction
  arc A93 (15.6157, -47.8698) -> (16.5757, -47.1665) centre (13.1605, -43.5112) ccw construction
  arc A94 (15.7035, -48.2189) -> (15.6157, -47.8698) centre (8.9947, -49.7216) ccw construction
  arc A95 (16.8821, -48.3839) -> (15.7035, -48.2189) centre (15.6039, -53.2204) ccw construction
  arc A96 (16.9413, -48.7985) -> (16.8821, -48.3839) centre (8.9947, -49.7216) ccw construction
  arc A97 (15.856, -49.2868) -> (16.9413, -48.7985) centre (14.3607, -44.513) ccw construction
  arc A98 (15.8693, -49.6465) -> (15.856, -49.2868) centre (8.9947, -49.7216) ccw construction
  arc A99 (16.9879, -50.053) -> (15.8693, -49.6465) centre (14.7321, -54.5181) ccw construction
  arc A100 (16.9596, -50.4709) -> (16.9879, -50.053) centre (8.9947, -49.7216) ccw construction
  arc A101 (15.7964, -50.7229) -> (16.9596, -50.4709) centre (15.3264, -45.7425) ccw construction
  arc A102 (15.7347, -51.0775) -> (15.7964, -50.7229) centre (8.9947, -49.7216) ccw construction
  arc A103 (16.7443, -51.7076) -> (15.7347, -51.0775) centre (13.6095, -55.6061) ccw construction
  arc A104 (16.6297, -52.1105) -> (16.7443, -51.7076) centre (8.9947, -49.7216) ccw construction
  arc A105 (15.4396, -52.1151) -> (16.6297, -52.1105) centre (16.0153, -47.1458) ccw construction
  arc A106 (15.3055, -52.4492) -> (15.4396, -52.1151) centre (8.9947, -49.7216) ccw construction
  arc A107 (16.162, -53.2755) -> (15.3055, -52.4492) centre (12.2852, -56.437) ccw construction
  arc A108 (15.9662, -53.6457) -> (16.162, -53.2755) centre (8.9947, -49.7216) ccw construction
  arc A109 (14.8012, -53.4028) -> (15.9662, -53.6457) centre (16.3974, -48.6618) ccw construction
  arc A110 (14.6005, -53.7016) -> (14.8012, -53.4028) centre (8.9947, -49.7216) ccw construction
  arc A111 (15.2665, -54.688) -> (14.6005, -53.7016) centre (10.817, -56.9744) ccw construction
  arc A112 (14.998, -55.0094) -> (15.2665, -54.688) centre (8.9947, -49.7216) ccw construction
  arc A113 (13.9089, -54.5296) -> (14.998, -55.0094) centre (16.456, -50.224) ccw construction
  arc A114 (13.6505, -54.7802) -> (13.9089, -54.5296) centre (8.9947, -49.7216) ccw construction
  arc A115 (14.0969, -55.8834) -> (13.6505, -54.7802) centre (9.2693, -57.1947) ccw construction
  arc A116 (13.7674, -56.142) -> (14.0969, -55.8834) centre (8.9947, -49.7216) ccw construction
  arc A117 (12.8019, -55.4462) -> (13.7674, -56.142) centre (16.1885, -51.7644) ccw construction
  arc A118 (12.4971, -55.6376) -> (12.8019, -55.4462) centre (8.9947, -49.7216) ccw construction
  arc A119 (12.7043, -56.8096) -> (12.4971, -55.6376) centre (7.7095, -57.0885) ccw construction
  arc A120 (12.3283, -56.994) -> (12.7043, -56.8096) centre (8.9947, -49.7216) ccw construction
  arc A121 (19.3741, -44.9537) -> (18.7931, -43.649) centre (13.6387, -46.7262) ccw construction
  arc A122 (18.9897, -45.2774) -> (19.3741, -44.9537) centre (13, -37.7752) ccw construction
  arc A123 (17.8029, -44.483) -> (18.9897, -45.2774) centre (21.712, -39.9271) ccw construction
  arc A124 (17.4452, -44.7251) -> (17.8029, -44.483) centre (13, -37.7752) ccw construction
  arc A125 (17.7423, -46.122) -> (17.4452, -44.7251) centre (11.7637, -46.6634) ccw construction
  arc A126 (17.299, -46.3588) -> (17.7423, -46.122) centre (13, -37.7752) ccw construction
  arc A127 (16.3033, -45.335) -> (17.299, -46.3588) centre (21.0742, -41.6914) ccw construction
  arc A128 (15.9031, -45.4975) -> (16.3033, -45.335) centre (13, -37.7752) ccw construction
  arc A129 (15.9033, -46.9256) -> (15.9031, -45.4975) centre (9.9428, -46.2121) ccw construction
  arc A130 (15.4204, -47.065) -> (15.9033, -46.9256) centre (13, -37.7752) ccw construction
  arc A131 (14.6593, -45.8566) -> (15.4204, -47.065) centre (20.0835, -43.2845) ccw construction
  arc A132 (14.2341, -45.9323) -> (14.6593, -45.8566) centre (13, -37.7752) ccw construction
  arc A133 (13.9373, -47.3293) -> (14.2341, -45.9323) centre (8.2554, -45.3921) ccw construction
  arc A134 (13.436, -47.3652) -> (13.9373, -47.3293) centre (13, -37.7752) ccw construction
  arc A135 (12.9429, -46.025) -> (13.436, -47.3652) centre (18.7832, -44.6369) ccw construction
  arc A136 (12.5112, -46.0107) -> (12.9429, -46.025) centre (13, -37.7752) ccw construction
  arc A137 (11.9304, -47.3154) -> (12.5112, -46.0107) centre (6.7755, -44.2392) ccw construction
  arc A138 (11.4326, -47.2463) -> (11.9304, -47.3154) centre (13, -37.7752) ccw construction
  arc A139 (11.2289, -45.8328) -> (11.4326, -47.2463) centre (17.2302, -45.6893) ccw construction
  arc A140 (10.8096, -45.7291) -> (11.2289, -45.8328) centre (13, -37.7752) ccw construction
  arc A141 (9.9703, -46.8845) -> (10.8096, -45.7291) centre (5.5675, -42.8038) ccw construction
  arc A142 (9.4977, -46.7135) -> (9.9703, -46.8845) centre (13, -37.7752) ccw construction
  arc A143 (9.5923, -45.2885) -> (9.4977, -46.7135) centre (15.4923, -46.3959) ccw construction
  arc A144 (9.2038, -45.0998) -> (9.5923, -45.2885) centre (13, -37.7752) ccw construction
  arc A145 (8.1425, -46.0556) -> (9.2038, -45.0998) centre (4.6844, -41.1486) ccw construction
  arc A146 (7.7158, -45.79) -> (8.1425, -46.0556) centre (13, -37.7752) ccw construction
  arc A147 (8.1047, -44.4158) -> (7.7158, -45.79) centre (13.6455, -46.7257) ccw construction
  arc A148 (7.7638, -44.1505) -> (8.1047, -44.4158) centre (13, -37.7752) ccw construction
  arc A149 (6.5271, -44.8647) -> (7.7638, -44.1505) centre (4.1648, -39.346) ccw construction
  arc A150 (6.1649, -44.5162) -> (6.5271, -44.8647) centre (13, -37.7752) ccw construction
  arc A151 (6.831, -43.2529) -> (6.1649, -44.5162) centre (11.7705, -46.6643) ccw construction
  arc A152 (6.5527, -42.9225) -> (6.831, -43.2529) centre (13, -37.7752) ccw construction
  arc A153 (5.1945, -43.364) -> (6.5527, -42.9225) centre (4.0312, -37.4747) ccw construction
  arc A154 (4.9127, -42.9478) -> (5.1945, -43.364) centre (13, -37.7752) ccw construction
  arc A155 (5.8269, -41.8506) -> (4.9127, -42.9478) centre (9.9492, -46.2144) ccw construction
  arc A156 (5.6234, -41.4696) -> (5.8269, -41.8506) centre (13, -37.7752) ccw construction
  arc A157 (4.2031, -41.619) -> (5.6234, -41.4696) centre (4.2897, -35.6166) ccw construction
  arc A158 (4.014, -41.1533) -> (4.2031, -41.619) centre (13, -37.7752) ccw construction
  arc A159 (5.1363, -40.2701) -> (4.014, -41.1533) centre (8.2612, -45.3957) ccw construction
  arc A160 (5.0165, -39.8552) -> (5.1363, -40.2701) centre (13, -37.7752) ccw construction
  arc A161 (3.5962, -39.706) -> (5.0165, -39.8552) centre (4.9288, -33.8528) ccw construction
  arc A162 (3.508, -39.2112) -> (3.5962, -39.706) centre (13, -37.7752) ccw construction
  arc A163 (4.7894, -38.5807) -> (3.508, -39.2112) centre (6.7804, -44.2439) ccw construction
  arc A164 (4.7585, -38.1499) -> (4.7894, -38.5807) centre (13, -37.7752) ccw construction
  arc A165 (3.4002, -37.7087) -> (4.7585, -38.1499) centre (5.9207, -32.2604) ccw construction
  arc A166 (3.4169, -37.2063) -> (3.4002, -37.7087) centre (13, -37.7752) ccw construction
  arc A167 (4.8014, -36.856) -> (3.4169, -37.2063) centre (5.5713, -42.8095) ccw construction
  arc A168 (4.8607, -36.4282) -> (4.8014, -36.856) centre (13, -37.7752) ccw construction
  arc A169 (3.6238, -35.7142) -> (4.8607, -36.4282) centre (7.222, -30.909) ccw construction
  arc A170 (3.7445, -35.2263) -> (3.6238, -35.7142) centre (13, -37.7752) ccw construction
  arc A171 (5.1716, -35.1715) -> (3.7445, -35.2263) centre (4.687, -41.1549) ccw construction
  arc A172 (5.3186, -34.7653) -> (5.1716, -35.1715) centre (13, -37.7752) ccw construction
  arc A173 (4.2572, -33.8098) -> (5.3186, -34.7653) centre (8.7758, -29.8578) ccw construction
  arc A174 (4.4767, -33.3577) -> (4.2572, -33.8098) centre (13, -37.7752) ccw construction
  arc A175 (5.884, -33.6008) -> (4.4767, -33.3577) centre (4.1659, -39.3527) ccw construction
  arc A176 (6.1122, -33.2341) -> (5.884, -33.6008) centre (13, -37.7752) ccw construction
  arc A177 (5.2727, -32.0788) -> (6.1122, -33.2341) centre (10.5142, -29.1525) ccw construction
  arc A178 (5.5814, -31.6822) -> (5.2727, -32.0788) centre (13, -37.7752) ccw construction
  arc A179 (6.9074, -32.2125) -> (5.5814, -31.6822) centre (4.031, -37.4815) ccw construction
  arc A180 (7.2069, -31.9013) -> (6.9074, -32.2125) centre (13, -37.7752) ccw construction
  arc A181 (6.6259, -30.5966) -> (7.2069, -31.9013) centre (12.3613, -28.8241) ccw construction
  arc A182 (7.0103, -30.2729) -> (6.6259, -30.5966) centre (13, -37.7752) ccw construction
  arc A183 (8.1971, -31.0673) -> (7.0103, -30.2729) centre (4.288, -35.6232) ccw construction
  arc A184 (8.5548, -30.8252) -> (8.1971, -31.0673) centre (13, -37.7752) ccw construction
  arc A185 (8.2577, -29.4283) -> (8.5548, -30.8252) centre (14.2363, -28.8869) ccw construction
  arc A186 (8.701, -29.1915) -> (8.2577, -29.4283) centre (13, -37.7752) ccw construction
  arc A187 (9.6967, -30.2153) -> (8.701, -29.1915) centre (4.9258, -33.8589) ccw construction
  arc A188 (10.0969, -30.0528) -> (9.6967, -30.2153) centre (13, -37.7752) ccw construction
  arc A189 (10.0967, -28.6247) -> (10.0969, -30.0528) centre (16.0572, -29.3382) ccw construction
  arc A190 (10.5796, -28.4853) -> (10.0967, -28.6247) centre (13, -37.7752) ccw construction
  arc A191 (11.3407, -29.6937) -> (10.5796, -28.4853) centre (5.9165, -32.2658) ccw construction
  arc A192 (11.7659, -29.618) -> (11.3407, -29.6937) centre (13, -37.7752) ccw construction
  arc A193 (12.0627, -28.221) -> (11.7659, -29.618) centre (17.7446, -30.1582) ccw construction
  arc A194 (12.564, -28.1851) -> (12.0627, -28.221) centre (13, -37.7752) ccw construction
  arc A195 (13.0571, -29.5253) -> (12.564, -28.1851) centre (7.2168, -30.9134) ccw construction
  arc A196 (13.4888, -29.5396) -> (13.0571, -29.5253) centre (13, -37.7752) ccw construction
  arc A197 (14.0696, -28.2349) -> (13.4888, -29.5396) centre (19.2245, -31.3111) ccw construction
  arc A198 (14.5674, -28.304) -> (14.0696, -28.2349) centre (13, -37.7752) ccw construction
  arc A199 (14.7711, -29.7175) -> (14.5674, -28.304) centre (8.7698, -29.861) ccw construction
  arc A200 (15.1904, -29.8212) -> (14.7711, -29.7175) centre (13, -37.7752) ccw construction
  arc A201 (16.0297, -28.6658) -> (15.1904, -29.8212) centre (20.4325, -32.7465) ccw construction
  arc A202 (16.5023, -28.8368) -> (16.0297, -28.6658) centre (13, -37.7752) ccw construction
  arc A203 (16.4077, -30.2618) -> (16.5023, -28.8368) centre (10.5077, -29.1544) ccw construction
  arc A204 (16.7962, -30.4505) -> (16.4077, -30.2618) centre (13, -37.7752) ccw construction
  arc A205 (17.8575, -29.4947) -> (16.7962, -30.4505) centre (21.3156, -34.4017) ccw construction
  arc A206 (18.2842, -29.7603) -> (17.8575, -29.4947) centre (13, -37.7752) ccw construction
  arc A207 (17.8953, -31.1345) -> (18.2842, -29.7603) centre (12.3545, -28.8246) ccw construction
  arc A208 (18.2362, -31.3998) -> (17.8953, -31.1345) centre (13, -37.7752) ccw construction
  arc A209 (19.4729, -30.6856) -> (18.2362, -31.3998) centre (21.8352, -36.2043) ccw construction
  arc A210 (19.8351, -31.0341) -> (19.4729, -30.6856) centre (13, -37.7752) ccw construction
  arc A211 (19.169, -32.2974) -> (19.8351, -31.0341) centre (14.2295, -28.886) ccw construction
  arc A212 (19.4473, -32.6278) -> (19.169, -32.2974) centre (13, -37.7752) ccw construction
  arc A213 (20.8055, -32.1863) -> (19.4473, -32.6278) centre (21.9688, -38.0756) ccw construction
  arc A214 (21.0873, -32.6025) -> (20.8055, -32.1863) centre (13, -37.7752) ccw construction
  arc A215 (20.1731, -33.6997) -> (21.0873, -32.6025) centre (16.0508, -29.3359) ccw construction
  arc A216 (20.3766, -34.0807) -> (20.1731, -33.6997) centre (13, -37.7752) ccw construction
  arc A217 (21.7969, -33.9313) -> (20.3766, -34.0807) centre (21.7103, -39.9337) ccw construction
  arc A218 (21.986, -34.397) -> (21.7969, -33.9313) centre (13, -37.7752) ccw construction
  arc A219 (20.8637, -35.2802) -> (21.986, -34.397) centre (17.7388, -30.1546) ccw construction
  arc A220 (20.9835, -35.6951) -> (20.8637, -35.2802) centre (13, -37.7752) ccw construction
  arc A221 (22.4038, -35.8443) -> (20.9835, -35.6951) centre (21.0712, -41.6975) ccw construction
  arc A222 (22.492, -36.3391) -> (22.4038, -35.8443) centre (13, -37.7752) ccw construction
  arc A223 (21.2106, -36.9696) -> (22.492, -36.3391) centre (19.2196, -31.3064) ccw construction
  arc A224 (21.2415, -37.4004) -> (21.2106, -36.9696) centre (13, -37.7752) ccw construction
  arc A225 (22.5998, -37.8416) -> (21.2415, -37.4004) centre (20.0793, -43.2899) ccw construction
  arc A226 (22.5831, -38.344) -> (22.5998, -37.8416) centre (13, -37.7752) ccw projected
  arc A227 (21.1986, -38.6943) -> (22.5831, -38.344) centre (20.4287, -32.7408) ccw construction
  arc A228 (21.1393, -39.1221) -> (21.1986, -38.6943) centre (13, -37.7752) ccw construction
  arc A229 (22.3762, -39.8361) -> (21.1393, -39.1221) centre (18.778, -44.6413) ccw construction